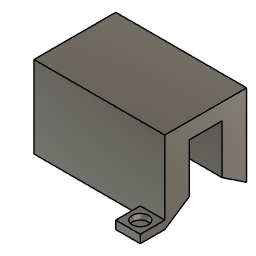
pied prin v1 (Autodesk Fusion 360 design; units mm, degrees)
Autodesk Fusion 360 part; units mm, degrees
note: some values were not read from the file. Set by a fixed rule: which sketch regions a step uses.
sketch "Esquisse1" plane through (0, 0, 0) normal (0, 0, 1) x (1, 0, 0)
  line L0 (0, 0) -> (100, 0)
  line L1 (100, 0) -> (100, 50)
  line L2 (100, 50) -> (0, 50)
  line L3 (0, 50) -> (0, 0)
  dimension "d1" = 100
  dimension "d2" = 50
  constraint horizontal L0
  constraint vertical L1
  constraint horizontal L2
  constraint vertical L3
  constraint coincident L0.start L3.end
  measures "d1" distance of L0.start L0.end
  measures "d2" distance of L0.start L2.end
extrude "Extrusion1" add sketch "Esquisse1" along normal blind 60
sketch "Esquisse2" plane through (0, 0, 0) normal (-1, 0, 0) x (0, -1, 0)
  line L0 (-50, 0) -> (0, 0)
  line L1 (0, 0) -> (0, 60)
  line L2 (0, 60) -> (-50, 60)
  line L3 (-50, 60) -> (-50, 0)
  line L4 (-35, 0) -> (-15, 0)
  line L5 (-15, 0) -> (-15, 40)
  line L6 (-15, 40) -> (-35, 40)
  line L7 (-35, 40) -> (-35, 0)
  dimension "d5" = 15
  dimension "d6" = 20
  dimension "d7" = 40
  constraint horizontal L4
  constraint vertical L5
  constraint horizontal L6
  constraint vertical L7
  constraint coincident L0 L4.start
  measures "d5" distance of L3 L7
  measures "d6" distance of L5.end L6.end
  measures "d7" distance of L4.end L5.end
extrude "Extrusion2" cut 1 faces at (33.3333, 33.3333, 60) along direction (0, 0, -1) blind 10
extrude "Extrusion3" cut sketch "Esquisse2" against normal blind 122 contours L0 L4 L5 L6 L7
extrude "Extrusion4" cut 1 faces at (100, 5, 30) along direction (-1, 0, 0) blind 20
sketch "Esquisse5" plane through (0, 0, 0) normal (-1, 0, 0) x (0, -1, 0)
  line L0 (-15, 40) -> (-15, 0)
  line L1 (-15, 0) -> (0, 0)
  line L2 (0, 0) -> (0, 50)
  line L3 (0, 50) -> (-50, 50)
  line L4 (-50, 50) -> (-50, 0)
  line L5 (-50, 0) -> (-35, 0)
  line L6 (-35, 0) -> (-35, 40)
  line L7 (-35, 40) -> (-15, 40)
  line L8 (-35, 0) -> (-35, 10)
  line L9 (-35, 10) -> (-50, 0)
  line L10 (-15, 0) -> (-15, 10)
  line L11 (-15, 10) -> (0, 0)
  dimension "d14" = 10
  dimension "d15" = 10
  constraint coincident L5.end L6.start
  constraint coincident L6 L8.end
  constraint coincident L4.end L5.start
  constraint coincident L0.end L1.start
  constraint perpendicular L1 L10
  constraint coincident L1.end L2.start
  measures "d14" distance of L5.end L8.end
  measures "d15" distance of L0.end L10.end
extrude "Extrusion5" cut sketch "Esquisse5" against normal blind 285 contours L0 L1 L10 L11 | L5 L6 L8 L9
sketch "Esquisse7" plane through (0, 0, 0) normal (0, -1, 0) x (1, 0, 0)
  line L0 (80, 0) -> (80, 50)
  line L1 (80, 50) -> (0, 50)
  line L2 (0, 50) -> (0, 0)
  line L3 (0, 0) -> (80, 0)
  line L4 (80, 0) -> (65, 0)
  line L5 (65, 0) -> (65, 5)
  line L6 (65, 5) -> (80, 5)
  line L7 (80, 5) -> (80, 0)
  dimension "d18" = 5
  dimension "d19" = 15
  constraint horizontal L4
  constraint vertical L5
  constraint horizontal L6
  constraint vertical L7
  constraint coincident L0.start L3.end
  measures "d18" distance of L0.start L6.end
  measures "d19" distance of L5.end L6.end
extrude "Extrusion6" add sketch "Esquisse7" along normal blind 15 contours L0 L3 L4 L5 L6 L7
sketch "Esquisse9" plane through (0, 0, 5) normal (0, 0, 1) x (-1, 0, 0)
  line L0 (-80, 0) -> (-65, 0)
  line L1 (-65, 0) -> (-65, 15)
  line L2 (-65, 15) -> (-80, 15)
  line L3 (-80, 15) -> (-80, 0)
  line L4 (-65, 0) -> (-80, 15)
  line L5 (-65, 15) -> (-80, 0)
  circle A0 centre (-72.5, 7.5) radius 5
  dimension "d22" = 10
  constraint coincident L0.end L1.start
  constraint coincident L2.end L3.start
  constraint coincident L1.end L2.start
  constraint coincident L0.start L3.end
  constraint midpoint L4 A0.centre
  measures "d22" diameter of A0
extrude "Extrusion7" cut sketch "Esquisse9" against normal blind 3.5 contours L4 L5 A0 | L4 L5 A0 | L4 L5 A0 | L4 L5 A0
